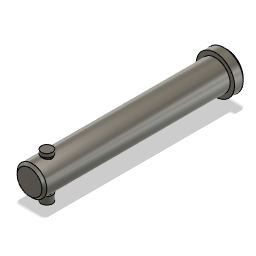
0.175.7694 - Axe d'articulation avec tête 12-75 type B (Autodesk Fusion 360 design; units mm, degrees)
Autodesk Fusion 360 part; units mm, degrees
sketch "Sketch1" plane through (0, 0, 0) normal (0, 0, 1) x (1, 0, 0)
  circle A0 centre (0, 0) radius 6
  dimension "d1" = 12
  constraint coincident A0.centre origin
  measures "d1" diameter of A0
extrude "Extrude1" add sketch "Sketch1" along normal blind 75 makes body 1
chamfer "Chamfer1" distance 1 angle 45 1 edges at (-5.594, -2.1697, 75) on bodies 1
sketch "Sketch2" plane through (0, 0, 0) normal (0, 0, -1) x (-1, 0, 0)
  circle A0 centre (0, 0) radius 6
  circle A1 centre (0, 0) radius 7.75
  dimension "d5" = 15.5
  constraint coincident A0.centre A1.centre
  measures "d5" diameter of A1
extrude "Extrude2" add sketch "Sketch2" along normal blind 4.5 contours A0 | A1 bodies 1
chamfer "Chamfer2" distance 1 angle 45 1 edges at (7.2255, -2.8025, -4.5) on bodies 1
sketch "Sketch3" plane through (0, 0, 0) normal (0, 1, 0) x (1, 0, 0)
  line L0 (-6, -74) -> (6, -74) construction
  line L1 (-6, -68) -> (6, -68) construction
  line L2 (0, -74) -> (0, -68) construction
  circle A0 centre (0, -68) radius 2
  dimension "d9" = 6
  dimension "d10" = 4
  constraint midpoint L0 L2.start
  constraint midpoint L1 L2.end
  constraint perpendicular L1 L2
  constraint coincident L2.end A0.centre
  measures "d10" diameter of A0
extrude "Extrude3" cut sketch "Sketch3" along normal through all and the other way through all bodies 1
sketch "Sketch4" plane through (0, 0, 0) normal (0, 1, 0) x (1, 0, 0)
  spline S0 degree 3 poles (2, -68) (2, -67.7467) (1.949, -67.478) (1.7443, -66.9859) (1.5907, -66.7623) (1.2378, -66.4093) (1.0142, -66.2557) (0.5219, -66.051) (0.2532, -66) (-0.2532, -66) (-0.5219, -66.051) (-1.0142, -66.2557) (-1.2378, -66.4093) (-1.5907, -66.7623) (-1.7443, -66.9859) (-1.949, -67.478) (-2, -67.7467) (-2, -68) (-2, -68.2533) (-1.949, -68.522) (-1.7443, -69.0141) (-1.5907, -69.2377) (-1.2378, -69.5907) (-1.0142, -69.7443) (-0.5219, -69.949) (-0.2532, -70) (0.2532, -70) (0.5219, -69.949) (1.0142, -69.7443) (1.2378, -69.5907) (1.5907, -69.2377) (1.7443, -69.0141) (1.949, -68.522) (2, -68.2533) (2, -68) knots 0.60776 0.60776 0.60776 0.60776 0.683748 0.683748 0.759735 0.759735 0.835688 0.835688 0.91164 0.91164 0.987593 0.987593 1.063545 1.063545 1.139533 1.139533 1.21552 1.21552 1.21552 1.291508 1.291508 1.367496 1.367496 1.443448 1.443448 1.5194 1.5194 1.595353 1.595353 1.671305 1.671305 1.747293 1.747293 1.82328 1.82328 1.82328 1.82328
  spline S1 degree 3 poles (-2, -68) (-2, -67.7467) (-1.949, -67.478) (-1.7443, -66.9859) (-1.5907, -66.7623) (-1.2378, -66.4093) (-1.0142, -66.2557) (-0.5219, -66.051) (-0.2532, -66) (0.2532, -66) (0.5219, -66.051) (1.0142, -66.2557) (1.2378, -66.4093) (1.5907, -66.7623) (1.7443, -66.9859) (1.949, -67.478) (2, -67.7467) (2, -68.2533) (1.949, -68.522) (1.7443, -69.0141) (1.5907, -69.2377) (1.2378, -69.5907) (1.0142, -69.7443) (0.5219, -69.949) (0.2532, -70) (-0.2532, -70) (-0.5219, -69.949) (-1.0142, -69.7443) (-1.2378, -69.5907) (-1.5907, -69.2377) (-1.7443, -69.0141) (-1.949, -68.522) (-2, -68.2533) (-2, -68) knots 0 0 0 0 0.075988 0.075988 0.151975 0.151975 0.227928 0.227928 0.30388 0.30388 0.379832 0.379832 0.455785 0.455785 0.531772 0.531772 0.60776 0.60776 0.683748 0.683748 0.759735 0.759735 0.835688 0.835688 0.91164 0.91164 0.987593 0.987593 1.063545 1.063545 1.139533 1.139533 1.21552 1.21552 1.21552 1.21552 construction
  spline S2 degree 3 poles (1.5, -68) (1.5, -67.8138) (1.4604, -67.6052) (1.385, -67.424) (1.3095, -67.2425) (1.1904, -67.0691) (1.0607, -66.9393) (0.931, -66.8096) (0.7575, -66.6905) (0.576, -66.615) (0.3947, -66.5396) (0.186, -66.5) (0, -66.5) (-0.186, -66.5) (-0.3947, -66.5396) (-0.576, -66.615) (-0.7575, -66.6905) (-0.931, -66.8096) (-1.0607, -66.9393) (-1.1904, -67.0691) (-1.3095, -67.2425) (-1.385, -67.424) (-1.4604, -67.6052) (-1.5, -67.8138) (-1.5, -68) (-1.5, -68.1862) (-1.4604, -68.3948) (-1.385, -68.576) (-1.3095, -68.7575) (-1.1904, -68.9309) (-1.0607, -69.0607) (-0.931, -69.1904) (-0.7575, -69.3095) (-0.576, -69.385) (-0.3947, -69.4604) (-0.186, -69.5) (0, -69.5) (0.186, -69.5) (0.3947, -69.4604) (0.576, -69.385) (0.7575, -69.3095) (0.931, -69.1904) (1.0607, -69.0607) (1.1904, -68.9309) (1.3095, -68.7575) (1.385, -68.576) (1.4604, -68.3948) (1.5, -68.1862) (1.5, -68) knots 0.60776 0.60776 0.60776 0.60776 0.683748 0.683748 0.683748 0.759735 0.759735 0.759735 0.835688 0.835688 0.835688 0.91164 0.91164 0.91164 0.987593 0.987593 0.987593 1.063545 1.063545 1.063545 1.139533 1.139533 1.139533 1.21552 1.21552 1.21552 1.291508 1.291508 1.291508 1.367496 1.367496 1.367496 1.443448 1.443448 1.443448 1.5194 1.5194 1.5194 1.595353 1.595353 1.595353 1.671305 1.671305 1.671305 1.747293 1.747293 1.747293 1.82328 1.82328 1.82328 1.82328
  dimension "d13" = 0.5
  measures "d13" distance of S0
extrude "Extrude4" add sketch "Sketch4" along normal blind 8 and the other way blind 10 separate body contours S2 makes body 2
sketch "Sketch5" plane through (0, 8, 0) normal (0, 1, 0) x (-1, 0, 0)
  spline S0 degree 3 poles (2, -68) (2, -67.7467) (1.949, -67.478) (1.7443, -66.9859) (1.5907, -66.7623) (1.2378, -66.4093) (1.0142, -66.2557) (0.5219, -66.051) (0.2532, -66) (-0.2532, -66) (-0.5219, -66.051) (-1.0142, -66.2557) (-1.2378, -66.4093) (-1.5907, -66.7623) (-1.7443, -66.9859) (-1.949, -67.478) (-2, -67.7467) (-2, -68) (-2, -68.2533) (-1.949, -68.522) (-1.7443, -69.0141) (-1.5907, -69.2377) (-1.2378, -69.5907) (-1.0142, -69.7443) (-0.5219, -69.949) (-0.2532, -70) (0.2532, -70) (0.5219, -69.949) (1.0142, -69.7443) (1.2378, -69.5907) (1.5907, -69.2377) (1.7443, -69.0141) (1.949, -68.522) (2, -68.2533) (2, -68) knots 0.60776 0.60776 0.60776 0.60776 0.683748 0.683748 0.759735 0.759735 0.835688 0.835688 0.91164 0.91164 0.987593 0.987593 1.063545 1.063545 1.139533 1.139533 1.21552 1.21552 1.21552 1.291508 1.291508 1.367496 1.367496 1.443448 1.443448 1.5194 1.5194 1.595353 1.595353 1.671305 1.671305 1.747293 1.747293 1.82328 1.82328 1.82328 1.82328
  spline S1 degree 3 poles (-2, -68) (-2, -67.7467) (-1.949, -67.478) (-1.7443, -66.9859) (-1.5907, -66.7623) (-1.2378, -66.4093) (-1.0142, -66.2557) (-0.5219, -66.051) (-0.2532, -66) (0.2532, -66) (0.5219, -66.051) (1.0142, -66.2557) (1.2378, -66.4093) (1.5907, -66.7623) (1.7443, -66.9859) (1.949, -67.478) (2, -67.7467) (2, -68.2533) (1.949, -68.522) (1.7443, -69.0141) (1.5907, -69.2377) (1.2378, -69.5907) (1.0142, -69.7443) (0.5219, -69.949) (0.2532, -70) (-0.2532, -70) (-0.5219, -69.949) (-1.0142, -69.7443) (-1.2378, -69.5907) (-1.5907, -69.2377) (-1.7443, -69.0141) (-1.949, -68.522) (-2, -68.2533) (-2, -68) knots 0 0 0 0 0.075988 0.075988 0.151975 0.151975 0.227928 0.227928 0.30388 0.30388 0.379832 0.379832 0.455785 0.455785 0.531772 0.531772 0.60776 0.60776 0.683748 0.683748 0.759735 0.759735 0.835688 0.835688 0.91164 0.91164 0.987593 0.987593 1.063545 1.063545 1.139533 1.139533 1.21552 1.21552 1.21552 1.21552 construction
  spline S2 degree 3 poles (1.5, -68) (1.5, -67.8138) (1.4604, -67.6052) (1.385, -67.424) (1.3095, -67.2425) (1.1904, -67.0691) (1.0607, -66.9393) (0.931, -66.8096) (0.7575, -66.6905) (0.576, -66.615) (0.3947, -66.5396) (0.186, -66.5) (0, -66.5) (-0.186, -66.5) (-0.3947, -66.5396) (-0.576, -66.615) (-0.7575, -66.6905) (-0.931, -66.8096) (-1.0607, -66.9393) (-1.1904, -67.0691) (-1.3095, -67.2425) (-1.385, -67.424) (-1.4604, -67.6052) (-1.5, -67.8138) (-1.5, -68) (-1.5, -68.1862) (-1.4604, -68.3948) (-1.385, -68.576) (-1.3095, -68.7575) (-1.1904, -68.9309) (-1.0607, -69.0607) (-0.931, -69.1904) (-0.7575, -69.3095) (-0.576, -69.385) (-0.3947, -69.4604) (-0.186, -69.5) (0, -69.5) (0.186, -69.5) (0.3947, -69.4604) (0.576, -69.385) (0.7575, -69.3095) (0.931, -69.1904) (1.0607, -69.0607) (1.1904, -68.9309) (1.3095, -68.7575) (1.385, -68.576) (1.4604, -68.3948) (1.5, -68.1862) (1.5, -68) knots 0.60776 0.60776 0.60776 0.60776 0.683748 0.683748 0.683748 0.759735 0.759735 0.759735 0.835688 0.835688 0.835688 0.91164 0.91164 0.91164 0.987593 0.987593 0.987593 1.063545 1.063545 1.063545 1.139533 1.139533 1.139533 1.21552 1.21552 1.21552 1.291508 1.291508 1.291508 1.367496 1.367496 1.367496 1.443448 1.443448 1.443448 1.5194 1.5194 1.5194 1.595353 1.595353 1.595353 1.671305 1.671305 1.671305 1.747293 1.747293 1.747293 1.82328 1.82328 1.82328 1.82328
  spline S3 degree 3 poles (-1.5, 68) (-1.5, 67.8138) (-1.4604, 67.6052) (-1.385, 67.424) (-1.3095, 67.2425) (-1.1904, 67.0691) (-1.0607, 66.9393) (-0.931, 66.8096) (-0.7575, 66.6905) (-0.576, 66.615) (-0.3947, 66.5396) (-0.186, 66.5) (0, 66.5) (0.186, 66.5) (0.3947, 66.5396) (0.576, 66.615) (0.7575, 66.6905) (0.931, 66.8096) (1.0607, 66.9393) (1.1904, 67.0691) (1.3095, 67.2425) (1.385, 67.424) (1.4604, 67.6052) (1.5, 67.8138) (1.5, 68) (1.5, 68.1862) (1.4604, 68.3948) (1.385, 68.576) (1.3095, 68.7575) (1.1904, 68.9309) (1.0607, 69.0607) (0.931, 69.1904) (0.7575, 69.3095) (0.576, 69.385) (0.3947, 69.4604) (0.186, 69.5) (0, 69.5) (-0.186, 69.5) (-0.3947, 69.4604) (-0.576, 69.385) (-0.7575, 69.3095) (-0.931, 69.1904) (-1.0607, 69.0607) (-1.1904, 68.9309) (-1.3095, 68.7575) (-1.385, 68.576) (-1.4604, 68.3948) (-1.5, 68.1862) (-1.5, 68) knots 0.60776 0.60776 0.60776 0.60776 0.683748 0.683748 0.683748 0.759735 0.759735 0.759735 0.835688 0.835688 0.835688 0.91164 0.91164 0.91164 0.987593 0.987593 0.987593 1.063545 1.063545 1.063545 1.139533 1.139533 1.139533 1.21552 1.21552 1.21552 1.291508 1.291508 1.291508 1.367496 1.367496 1.367496 1.443448 1.443448 1.443448 1.5194 1.5194 1.5194 1.595353 1.595353 1.595353 1.671305 1.671305 1.671305 1.747293 1.747293 1.747293 1.82328 1.82328 1.82328 1.82328 construction
  spline S4 degree 3 poles (-1.5, 68) (-1.5, 68.1862) (-1.4604, 68.3948) (-1.385, 68.576) (-1.3095, 68.7575) (-1.1904, 68.9309) (-1.0607, 69.0607) (-0.931, 69.1904) (-0.7575, 69.3095) (-0.576, 69.385) (-0.3947, 69.4604) (-0.186, 69.5) (0, 69.5) (0.186, 69.5) (0.3947, 69.4604) (0.576, 69.385) (0.7575, 69.3095) (0.931, 69.1904) (1.0607, 69.0607) (1.1904, 68.9309) (1.3095, 68.7575) (1.385, 68.576) (1.4604, 68.3948) (1.5, 68.1862) (1.5, 68) (1.5, 67.8138) (1.4604, 67.6052) (1.385, 67.424) (1.3095, 67.2425) (1.1904, 67.0691) (1.0607, 66.9393) (0.931, 66.8096) (0.7575, 66.6905) (0.576, 66.615) (0.3947, 66.5396) (0.186, 66.5) (0, 66.5) (-0.186, 66.5) (-0.3947, 66.5396) (-0.576, 66.615) (-0.7575, 66.6905) (-0.931, 66.8096) (-1.0607, 66.9393) (-1.1904, 67.0691) (-1.3095, 67.2425) (-1.385, 67.424) (-1.4604, 67.6052) (-1.5, 67.8138) (-1.5, 68) knots -1.82328 -1.82328 -1.82328 -1.82328 -1.747293 -1.747293 -1.747293 -1.671305 -1.671305 -1.671305 -1.595353 -1.595353 -1.595353 -1.5194 -1.5194 -1.5194 -1.443448 -1.443448 -1.443448 -1.367496 -1.367496 -1.367496 -1.291508 -1.291508 -1.291508 -1.21552 -1.21552 -1.21552 -1.139533 -1.139533 -1.139533 -1.063545 -1.063545 -1.063545 -0.987593 -0.987593 -0.987593 -0.91164 -0.91164 -0.91164 -0.835688 -0.835688 -0.835688 -0.759735 -0.759735 -0.759735 -0.683748 -0.683748 -0.683748 -0.60776 -0.60776 -0.60776 -0.60776 construction
  circle A0 centre (0, 68) radius 2.25
  spline S5 degree 3 poles (1.5, 68) (1.5, 68.1862) (1.4604, 68.3948) (1.385, 68.576) (1.3095, 68.7575) (1.1904, 68.9309) (1.0607, 69.0607) (0.931, 69.1904) (0.7575, 69.3095) (0.576, 69.385) (0.3947, 69.4604) (0.186, 69.5) (0, 69.5) (-0.186, 69.5) (-0.3947, 69.4604) (-0.576, 69.385) (-0.7575, 69.3095) (-0.931, 69.1904) (-1.0607, 69.0607) (-1.1904, 68.9309) (-1.3095, 68.7575) (-1.385, 68.576) (-1.4604, 68.3948) (-1.5, 68.1862) (-1.5, 68) (-1.5, 67.8138) (-1.4604, 67.6052) (-1.385, 67.424) (-1.3095, 67.2425) (-1.1904, 67.0691) (-1.0607, 66.9393) (-0.931, 66.8096) (-0.7575, 66.6905) (-0.576, 66.615) (-0.3947, 66.5396) (-0.186, 66.5) (0, 66.5) (0.186, 66.5) (0.3947, 66.5396) (0.576, 66.615) (0.7575, 66.6905) (0.931, 66.8096) (1.0607, 66.9393) (1.1904, 67.0691) (1.3095, 67.2425) (1.385, 67.424) (1.4604, 67.6052) (1.5, 67.8138) (1.5, 68) knots -1.82328 -1.82328 -1.82328 -1.82328 -1.747293 -1.747293 -1.747293 -1.671305 -1.671305 -1.671305 -1.595353 -1.595353 -1.595353 -1.5194 -1.5194 -1.5194 -1.443448 -1.443448 -1.443448 -1.367496 -1.367496 -1.367496 -1.291508 -1.291508 -1.291508 -1.21552 -1.21552 -1.21552 -1.139533 -1.139533 -1.139533 -1.063545 -1.063545 -1.063545 -0.987593 -0.987593 -0.987593 -0.91164 -0.91164 -0.91164 -0.835688 -0.835688 -0.835688 -0.759735 -0.759735 -0.759735 -0.683748 -0.683748 -0.683748 -0.60776 -0.60776 -0.60776 -0.60776 construction
  spline S6 degree 3 poles (1.5, 68) (1.4997, 68.0291) (1.499, 68.0582) (1.4876, 68.2407) (1.4443, 68.4464) (1.2744, 68.8221) (1.1579, 68.9635) (1.0607, 69.0607) (0.9778, 69.1435) (0.881, 69.2184) (0.6163, 69.3807) (0.5167, 69.4099) (0.2655, 69.4873) (0.0596, 69.5123) (-0.2987, 69.4775) (-0.5139, 69.4246) (-0.8641, 69.2393) (-1.0281, 69.1108) (-1.2584, 68.8304) (-1.3708, 68.6429) (-1.4869, 68.2672) (-1.5123, 68.0612) (-1.478, 67.7046) (-1.4256, 67.4888) (-1.2414, 67.1391) (-1.1133, 66.9745) (-0.8077, 66.7224) (-0.6295, 66.6258) (-0.2761, 66.5151) (-0.0693, 66.488) (0.2839, 66.5201) (0.5004, 66.5708) (0.8431, 66.7475) (1.0118, 66.8739) (1.2827, 67.1947) (1.368, 67.3621) (1.4579, 67.6311) (1.4977, 67.8165) (1.5, 68) knots -0.080744 -0.080744 -0.080744 -0.080744 -0.074519 -0.074519 -0.041241 -0.041241 0 0 0 0.035143 0.035143 0.092639 0.092639 0.246463 0.246463 0.37223 0.37223 0.489793 0.489793 0.586811 0.586811 0.67816 0.67816 0.752062 0.752062 0.820566 0.820566 0.888592 0.888592 0.958337 0.958337 1.013363 1.013363 1.062684 1.062684 1.116599 1.116599 1.155794 1.155794 1.155794 1.155794 construction
  spline S7 degree 3 poles (1.5, 68) (1.5, 68.1862) (1.4604, 68.3948) (1.385, 68.576) (1.3095, 68.7575) (1.1904, 68.9309) (1.0607, 69.0607) (0.931, 69.1904) (0.7575, 69.3095) (0.576, 69.385) (0.3947, 69.4604) (0.186, 69.5) (0, 69.5) (-0.186, 69.5) (-0.3947, 69.4604) (-0.576, 69.385) (-0.7575, 69.3095) (-0.931, 69.1904) (-1.0607, 69.0607) (-1.1904, 68.9309) (-1.3095, 68.7575) (-1.385, 68.576) (-1.4604, 68.3948) (-1.5, 68.1862) (-1.5, 68) (-1.5, 67.8138) (-1.4604, 67.6052) (-1.385, 67.424) (-1.3095, 67.2425) (-1.1904, 67.0691) (-1.0607, 66.9393) (-0.931, 66.8096) (-0.7575, 66.6905) (-0.576, 66.615) (-0.3947, 66.5396) (-0.186, 66.5) (0, 66.5) (0.186, 66.5) (0.3947, 66.5396) (0.576, 66.615) (0.7575, 66.6905) (0.931, 66.8096) (1.0607, 66.9393) (1.1904, 67.0691) (1.3095, 67.2425) (1.385, 67.424) (1.4604, 67.6052) (1.5, 67.8138) (1.5, 68) knots -1.82328 -1.82328 -1.82328 -1.82328 -1.747293 -1.747293 -1.747293 -1.671305 -1.671305 -1.671305 -1.595353 -1.595353 -1.595353 -1.5194 -1.5194 -1.5194 -1.443448 -1.443448 -1.443448 -1.367496 -1.367496 -1.367496 -1.291508 -1.291508 -1.291508 -1.21552 -1.21552 -1.21552 -1.139533 -1.139533 -1.139533 -1.063545 -1.063545 -1.063545 -0.987593 -0.987593 -0.987593 -0.91164 -0.91164 -0.91164 -0.835688 -0.835688 -0.835688 -0.759735 -0.759735 -0.759735 -0.683748 -0.683748 -0.683748 -0.60776 -0.60776 -0.60776 -0.60776 construction
  spline S8 degree 3 poles (2, 68) (2, 67.7467) (1.949, 67.478) (1.7443, 66.9859) (1.5907, 66.7623) (1.2378, 66.4093) (1.0142, 66.2557) (0.5219, 66.051) (0.2532, 66) (-0.2532, 66) (-0.5219, 66.051) (-1.0142, 66.2557) (-1.2378, 66.4093) (-1.5907, 66.7623) (-1.7443, 66.9859) (-1.949, 67.478) (-2, 67.7467) (-2, 68) (-2, 68.2533) (-1.949, 68.522) (-1.7443, 69.0141) (-1.5907, 69.2377) (-1.2378, 69.5907) (-1.0142, 69.7443) (-0.5219, 69.949) (-0.2532, 70) (0.2532, 70) (0.5219, 69.949) (1.0142, 69.7443) (1.2378, 69.5907) (1.5907, 69.2377) (1.7443, 69.0141) (1.949, 68.522) (2, 68.2533) (2, 68) knots 0.60776 0.60776 0.60776 0.60776 0.683748 0.683748 0.759735 0.759735 0.835688 0.835688 0.91164 0.91164 0.987593 0.987593 1.063545 1.063545 1.139533 1.139533 1.21552 1.21552 1.21552 1.291508 1.291508 1.367496 1.367496 1.443448 1.443448 1.5194 1.5194 1.595353 1.595353 1.671305 1.671305 1.747293 1.747293 1.82328 1.82328 1.82328 1.82328
  spline S9 degree 3 poles (-2, 68) (-2, 67.7467) (-1.949, 67.478) (-1.7443, 66.9859) (-1.5907, 66.7623) (-1.2378, 66.4093) (-1.0142, 66.2557) (-0.5219, 66.051) (-0.2532, 66) (0.2532, 66) (0.5219, 66.051) (1.0142, 66.2557) (1.2378, 66.4093) (1.5907, 66.7623) (1.7443, 66.9859) (1.949, 67.478) (2, 67.7467) (2, 68.2533) (1.949, 68.522) (1.7443, 69.0141) (1.5907, 69.2377) (1.2378, 69.5907) (1.0142, 69.7443) (0.5219, 69.949) (0.2532, 70) (-0.2532, 70) (-0.5219, 69.949) (-1.0142, 69.7443) (-1.2378, 69.5907) (-1.5907, 69.2377) (-1.7443, 69.0141) (-1.949, 68.522) (-2, 68.2533) (-2, 68) knots 0 0 0 0 0.075988 0.075988 0.151975 0.151975 0.227928 0.227928 0.30388 0.30388 0.379832 0.379832 0.455785 0.455785 0.531772 0.531772 0.60776 0.60776 0.683748 0.683748 0.759735 0.759735 0.835688 0.835688 0.91164 0.91164 0.987593 0.987593 1.063545 1.063545 1.139533 1.139533 1.21552 1.21552 1.21552 1.21552 construction
  dimension "d18" = 4.5
  measures "d13" distance of S0
  measures "d18" diameter of A0
extrude "Extrude5" add sketch "Sketch5" against normal blind 1.5 contours A0 | S8 bodies 2
sketch "Sketch6" plane through (0, -10, 0) normal (0, -1, 0) x (1, 0, 0)
  spline S0 degree 3 poles (1.5, 68) (1.5, 68.1862) (1.4604, 68.3948) (1.385, 68.576) (1.3095, 68.7575) (1.1904, 68.9309) (1.0607, 69.0607) (0.931, 69.1904) (0.7575, 69.3095) (0.576, 69.385) (0.3947, 69.4604) (0.186, 69.5) (0, 69.5) (-0.186, 69.5) (-0.3947, 69.4604) (-0.576, 69.385) (-0.7575, 69.3095) (-0.931, 69.1904) (-1.0607, 69.0607) (-1.1904, 68.9309) (-1.3095, 68.7575) (-1.385, 68.576) (-1.4604, 68.3948) (-1.5, 68.1862) (-1.5, 68) (-1.5, 67.8138) (-1.4604, 67.6052) (-1.385, 67.424) (-1.3095, 67.2425) (-1.1904, 67.0691) (-1.0607, 66.9393) (-0.931, 66.8096) (-0.7575, 66.6905) (-0.576, 66.615) (-0.3947, 66.5396) (-0.186, 66.5) (0, 66.5) (0.186, 66.5) (0.3947, 66.5396) (0.576, 66.615) (0.7575, 66.6905) (0.931, 66.8096) (1.0607, 66.9393) (1.1904, 67.0691) (1.3095, 67.2425) (1.385, 67.424) (1.4604, 67.6052) (1.5, 67.8138) (1.5, 68) knots -1.82328 -1.82328 -1.82328 -1.82328 -1.747293 -1.747293 -1.747293 -1.671305 -1.671305 -1.671305 -1.595353 -1.595353 -1.595353 -1.5194 -1.5194 -1.5194 -1.443448 -1.443448 -1.443448 -1.367496 -1.367496 -1.367496 -1.291508 -1.291508 -1.291508 -1.21552 -1.21552 -1.21552 -1.139533 -1.139533 -1.139533 -1.063545 -1.063545 -1.063545 -0.987593 -0.987593 -0.987593 -0.91164 -0.91164 -0.91164 -0.835688 -0.835688 -0.835688 -0.759735 -0.759735 -0.759735 -0.683748 -0.683748 -0.683748 -0.60776 -0.60776 -0.60776 -0.60776 construction
  spline S1 degree 3 poles (1.5, 68) (1.4997, 68.0291) (1.499, 68.0582) (1.4876, 68.2407) (1.4443, 68.4464) (1.2744, 68.8221) (1.1579, 68.9635) (1.0607, 69.0607) (0.9778, 69.1435) (0.881, 69.2184) (0.6163, 69.3807) (0.5167, 69.4099) (0.2655, 69.4873) (0.0596, 69.5123) (-0.2987, 69.4775) (-0.5139, 69.4246) (-0.8641, 69.2393) (-1.0281, 69.1108) (-1.2584, 68.8304) (-1.3708, 68.6429) (-1.4869, 68.2672) (-1.5123, 68.0612) (-1.478, 67.7046) (-1.4256, 67.4888) (-1.2414, 67.1391) (-1.1133, 66.9745) (-0.8077, 66.7224) (-0.6295, 66.6258) (-0.2761, 66.5151) (-0.0693, 66.488) (0.2839, 66.5201) (0.5004, 66.5708) (0.8431, 66.7475) (1.0118, 66.8739) (1.2827, 67.1947) (1.368, 67.3621) (1.4579, 67.6311) (1.4977, 67.8165) (1.5, 68) knots -0.080744 -0.080744 -0.080744 -0.080744 -0.074519 -0.074519 -0.041241 -0.041241 0 0 0 0.035143 0.035143 0.092639 0.092639 0.246463 0.246463 0.37223 0.37223 0.489793 0.489793 0.586811 0.586811 0.67816 0.67816 0.752062 0.752062 0.820566 0.820566 0.888592 0.888592 0.958337 0.958337 1.013363 1.013363 1.062684 1.062684 1.116599 1.116599 1.155794 1.155794 1.155794 1.155794 construction
  spline S2 degree 3 poles (1.5, 68) (1.5, 68.1862) (1.4604, 68.3948) (1.385, 68.576) (1.3095, 68.7575) (1.1904, 68.9309) (1.0607, 69.0607) (0.931, 69.1904) (0.7575, 69.3095) (0.576, 69.385) (0.3947, 69.4604) (0.186, 69.5) (0, 69.5) (-0.186, 69.5) (-0.3947, 69.4604) (-0.576, 69.385) (-0.7575, 69.3095) (-0.931, 69.1904) (-1.0607, 69.0607) (-1.1904, 68.9309) (-1.3095, 68.7575) (-1.385, 68.576) (-1.4604, 68.3948) (-1.5, 68.1862) (-1.5, 68) (-1.5, 67.8138) (-1.4604, 67.6052) (-1.385, 67.424) (-1.3095, 67.2425) (-1.1904, 67.0691) (-1.0607, 66.9393) (-0.931, 66.8096) (-0.7575, 66.6905) (-0.576, 66.615) (-0.3947, 66.5396) (-0.186, 66.5) (0, 66.5) (0.186, 66.5) (0.3947, 66.5396) (0.576, 66.615) (0.7575, 66.6905) (0.931, 66.8096) (1.0607, 66.9393) (1.1904, 67.0691) (1.3095, 67.2425) (1.385, 67.424) (1.4604, 67.6052) (1.5, 67.8138) (1.5, 68) knots -1.82328 -1.82328 -1.82328 -1.82328 -1.747293 -1.747293 -1.747293 -1.671305 -1.671305 -1.671305 -1.595353 -1.595353 -1.595353 -1.5194 -1.5194 -1.5194 -1.443448 -1.443448 -1.443448 -1.367496 -1.367496 -1.367496 -1.291508 -1.291508 -1.291508 -1.21552 -1.21552 -1.21552 -1.139533 -1.139533 -1.139533 -1.063545 -1.063545 -1.063545 -0.987593 -0.987593 -0.987593 -0.91164 -0.91164 -0.91164 -0.835688 -0.835688 -0.835688 -0.759735 -0.759735 -0.759735 -0.683748 -0.683748 -0.683748 -0.60776 -0.60776 -0.60776 -0.60776 construction
  spline S3 degree 3 poles (2, 68) (2, 67.7467) (1.949, 67.478) (1.7443, 66.9859) (1.5907, 66.7623) (1.2378, 66.4093) (1.0142, 66.2557) (0.5219, 66.051) (0.2532, 66) (-0.2532, 66) (-0.5219, 66.051) (-1.0142, 66.2557) (-1.2378, 66.4093) (-1.5907, 66.7623) (-1.7443, 66.9859) (-1.949, 67.478) (-2, 67.7467) (-2, 68) (-2, 68.2533) (-1.949, 68.522) (-1.7443, 69.0141) (-1.5907, 69.2377) (-1.2378, 69.5907) (-1.0142, 69.7443) (-0.5219, 69.949) (-0.2532, 70) (0.2532, 70) (0.5219, 69.949) (1.0142, 69.7443) (1.2378, 69.5907) (1.5907, 69.2377) (1.7443, 69.0141) (1.949, 68.522) (2, 68.2533) (2, 68) knots 0.60776 0.60776 0.60776 0.60776 0.683748 0.683748 0.759735 0.759735 0.835688 0.835688 0.91164 0.91164 0.987593 0.987593 1.063545 1.063545 1.139533 1.139533 1.21552 1.21552 1.21552 1.291508 1.291508 1.367496 1.367496 1.443448 1.443448 1.5194 1.5194 1.595353 1.595353 1.671305 1.671305 1.747293 1.747293 1.82328 1.82328 1.82328 1.82328
  spline S4 degree 3 poles (-2, 68) (-2, 67.7467) (-1.949, 67.478) (-1.7443, 66.9859) (-1.5907, 66.7623) (-1.2378, 66.4093) (-1.0142, 66.2557) (-0.5219, 66.051) (-0.2532, 66) (0.2532, 66) (0.5219, 66.051) (1.0142, 66.2557) (1.2378, 66.4093) (1.5907, 66.7623) (1.7443, 66.9859) (1.949, 67.478) (2, 67.7467) (2, 68.2533) (1.949, 68.522) (1.7443, 69.0141) (1.5907, 69.2377) (1.2378, 69.5907) (1.0142, 69.7443) (0.5219, 69.949) (0.2532, 70) (-0.2532, 70) (-0.5219, 69.949) (-1.0142, 69.7443) (-1.2378, 69.5907) (-1.5907, 69.2377) (-1.7443, 69.0141) (-1.949, 68.522) (-2, 68.2533) (-2, 68) knots 0 0 0 0 0.075988 0.075988 0.151975 0.151975 0.227928 0.227928 0.30388 0.30388 0.379832 0.379832 0.455785 0.455785 0.531772 0.531772 0.60776 0.60776 0.683748 0.683748 0.759735 0.759735 0.835688 0.835688 0.91164 0.91164 0.987593 0.987593 1.063545 1.063545 1.139533 1.139533 1.21552 1.21552 1.21552 1.21552 construction
  circle A0 centre (0, 68) radius 2.25
  dimension "d21" = 4.5
  measures "d21" diameter of A0
extrude "Extrude6" add sketch "Sketch6" against normal blind 3 contours S3 | A0 bodies 2
